Autodesk Inventor part; units mm, degrees
(part 3 of 3)
  spline S428 degree 2 poles (88.3492, 102.9904) (88.3492, 103.2264) (88.4685, 103.644) (88.7097, 103.9578) (89.0676, 104.1394) (89.3062, 104.1394) knots 0 0 0 1 2 3 4 4 4
  spline S429 degree 2 poles (89.3062, 104.1394) (89.3789, 104.1394) (89.5215, 104.1264) (89.5838, 104.1057) knots 0 0 0 1 2 2 2
  line L489 (89.5838, 104.1057) -> (89.7757, 103.8204)
  line L490 (89.7757, 103.8204) -> (89.7757, 104.1446)
  line L491 (89.7757, 104.1446) -> (90.1569, 104.1057)
  line L492 (90.1569, 104.1057) -> (90.1569, 101.8052)
  spline S430 degree 2 poles (90.1569, 101.8052) (90.1569, 101.6081) (90.0221, 101.2631) (89.7705, 101.0064) (89.4048, 100.8585) (89.1766, 100.8585) knots 0 0 0 1 2 3 4 4 4
  spline S431 degree 2 poles (89.1766, 100.8585) (89.0184, 100.8585) (88.7798, 100.9389) (88.6942, 100.9882) knots 0 0 0 1 2 2 2
  spline S432 degree 2 poles (88.6942, 100.9882) (88.5982, 101.0427) (88.5282, 101.1179) knots 0 0 0 1 1 1
  line L493 (88.5282, 101.1179) -> (88.7253, 101.3383)
  spline S433 degree 2 poles (88.7253, 101.3383) (88.7823, 101.2943) (88.855, 101.2579) knots 0 0 0 1 1 1
  spline S434 degree 2 poles (88.855, 101.2579) (88.9172, 101.2294) (89.0832, 101.1801) (89.1792, 101.1801) knots 0 0 0 1 2 2 2
  spline S435 degree 2 poles (89.1792, 101.1801) (89.3036, 101.1801) (89.5215, 101.2839) (89.6823, 101.4602) (89.7757, 101.6989) (89.7757, 101.8337) knots 0 0 0 1 2 3 4 4 4
  line L494 (89.7757, 101.8337) -> (89.7757, 102.1683)
  spline S436 degree 2 poles (89.7757, 103.5714) (89.7212, 103.6388) (89.6486, 103.6933) knots 0 0 0 1 1 1
  spline S437 degree 2 poles (89.6486, 103.6933) (89.5863, 103.74) (89.41, 103.8178) (89.2959, 103.8178) knots 0 0 0 1 2 2 2
  spline S438 degree 2 poles (89.2959, 103.8178) (89.174, 103.8178) (88.9976, 103.7426) (88.8705, 103.6129) (88.7927, 103.4417) (88.746, 103.2524) (88.7305, 103.0579) (88.7305, 102.9671) knots 0 0 0 1 2 3 4 5 6 6 6
  spline S439 degree 2 poles (88.7305, 102.9671) (88.7305, 102.7959) (88.8057, 102.5106) (88.9406, 102.3031) (89.1299, 102.1864) (89.244, 102.1864) knots 0 0 0 1 2 3 4 4 4
  spline S440 degree 2 poles (89.244, 102.1864) (89.3477, 102.1864) (89.5085, 102.2305) (89.6382, 102.3057) (89.7368, 102.3991) (89.7757, 102.4484) knots 0 0 0 1 2 3 4 4 4
  line L495 (89.7757, 102.4484) -> (89.7757, 103.5714)
  line L496 (92.1851, 104.1057) -> (92.5663, 104.1446)
  line L497 (92.5663, 104.1446) -> (92.5663, 101.896)
  line L498 (92.5663, 101.896) -> (92.1851, 101.896)
  line L499 (92.1851, 101.896) -> (92.1851, 102.2227)
  line L500 (92.1851, 102.2227) -> (92.0632, 102.0101)
  spline S441 degree 2 poles (92.0632, 102.0101) (92.0269, 101.9841) (91.9283, 101.9323) (91.8038, 101.8908) (91.656, 101.8622) (91.573, 101.8622) knots 0 0 0 1 2 3 4 4 4
  spline S442 degree 2 poles (91.573, 101.8622) (91.4122, 101.8622) (91.1814, 101.979) (91.0335, 102.1864) (90.9609, 102.4743) (90.9609, 102.6429) knots 0 0 0 1 2 3 4 4 4
  line L501 (90.9609, 102.6429) -> (90.9609, 104.1057)
  line L502 (90.9609, 104.1057) -> (91.3422, 104.1446)
  line L503 (91.3422, 104.1446) -> (91.3422, 102.6429)
  spline S443 degree 2 poles (91.3422, 102.6429) (91.3422, 102.4276) (91.5159, 102.1838) (91.7027, 102.1838) knots 0 0 0 1 2 2 2
  spline S444 degree 2 poles (91.7027, 102.1838) (91.7727, 102.1838) (91.905, 102.2279) (92.0295, 102.2954) (92.1384, 102.3758) (92.1851, 102.4147) knots 0 0 0 1 2 3 4 4 4
  line L504 (92.1851, 102.4147) -> (92.1851, 104.1057)
  line L505 (93.7516, 101.896) -> (93.3703, 101.896)
  line L506 (93.3703, 101.896) -> (93.3703, 104.0149)
  line L507 (93.3703, 104.0149) -> (93.7516, 104.0564)
  line L508 (93.7516, 104.0564) -> (93.7516, 101.896)
  line L509 (93.3573, 104.9071) -> (93.7645, 104.9071)
  line L510 (93.7645, 104.9071) -> (93.7645, 104.5051)
  line L511 (93.7645, 104.5051) -> (93.3573, 104.5051)
  line L512 (93.3573, 104.5051) -> (93.3573, 104.9071)
  line L513 (95.7979, 101.896) -> (95.7979, 102.2202)
  line L514 (95.7979, 102.2202) -> (95.6059, 101.9945)
  spline S445 degree 2 poles (95.6059, 101.9945) (95.5722, 101.9712) (95.4866, 101.9219) (95.3829, 101.8856) (95.2558, 101.8622) (95.178, 101.8622) knots 0 0 0 1 2 3 4 4 4
  spline S446 degree 2 poles (95.178, 101.8622) (95.012, 101.8622) (94.7267, 102.0256) (94.5167, 102.3135) (94.3948, 102.7129) (94.3948, 102.9515) knots 0 0 0 1 2 3 4 4 4
  spline S447 degree 2 poles (94.3948, 102.9515) (94.3948, 103.1927) (94.5504, 103.6129) (94.8357, 103.9241) (95.2377, 104.1031) (95.4866, 104.1031) knots 0 0 0 1 2 3 4 4 4
  line L515 (95.4866, 104.1031) -> (95.7979, 104.1031)
  line L516 (95.7979, 104.1031) -> (95.7979, 105.1483)
  line L517 (95.7979, 105.1483) -> (96.1791, 105.1094)
  line L518 (96.1791, 105.1094) -> (96.1791, 102.2565)
  line L519 (96.1791, 102.2565) -> (96.218, 101.896)
  line L520 (96.218, 101.896) -> (95.7979, 101.896)
  spline S448 degree 2 poles (95.4892, 103.7815) (95.3051, 103.7815) (95.0354, 103.644) (94.859, 103.408) (94.776, 103.0864) (94.776, 102.9048) knots 0 0 0 1 2 3 4 4 4
  spline S449 degree 2 poles (94.776, 102.9048) (94.776, 102.7259) (94.859, 102.4562) (94.9939, 102.2772) (95.1676, 102.1864) (95.2558, 102.1864) knots 0 0 0 1 2 3 4 4 4
  spline S450 degree 2 poles (95.2558, 102.1864) (95.3518, 102.1864) (95.5126, 102.2513) (95.65, 102.3472) (95.759, 102.4614) (95.7979, 102.5106) knots 0 0 0 1 2 3 4 4 4
  line L521 (95.7979, 102.5106) -> (95.7979, 103.7815)
  line L522 (95.7979, 103.7815) -> (95.4892, 103.7815)
  spline S451 degree 2 poles (98.5185, 102.1553) (98.4562, 102.0905) (98.3084, 101.9841) (98.1269, 101.9037) (97.909, 101.8622) (97.7741, 101.8622) knots 0 0 0 1 2 3 4 4 4
  spline S452 degree 2 poles (97.7741, 101.8622) (97.507, 101.8622) (97.1309, 102.0516) (96.8923, 102.368) (96.7808, 102.7778) (96.7808, 103.0008) knots 0 0 0 1 2 3 4 4 4
  spline S453 degree 2 poles (96.7808, 103.0008) (96.7808, 103.1435) (96.8327, 103.4236) (96.9364, 103.6751) (97.0946, 103.893) (97.3021, 104.0486) (97.5667, 104.1394) (97.7249, 104.1394) knots 0 0 0 1 2 3 4 5 6 6 6
  spline S454 degree 2 poles (97.7249, 104.1394) (97.9401, 104.1394) (98.2591, 103.9993) (98.4666, 103.7452) (98.5678, 103.3924) (98.5678, 103.1772) knots 0 0 0 1 2 3 4 4 4
  spline S455 degree 2 poles (98.5678, 103.1772) (98.5678, 103.1149) (98.56, 102.9671) (98.5522, 102.8997) knots 0 0 0 1 2 2 2
  line L523 (98.5522, 102.8997) -> (97.1621, 102.8997)
  spline S456 degree 2 poles (97.1621, 102.8997) (97.1621, 102.7492) (97.2451, 102.4899) (97.3929, 102.2954) (97.603, 102.1838) (97.7352, 102.1838) knots 0 0 0 1 2 3 4 4 4
  spline S457 degree 2 poles (97.7352, 102.1838) (97.8623, 102.1838) (98.0542, 102.2227) (98.1891, 102.2772) (98.2773, 102.3317) (98.3006, 102.3472) knots 0 0 0 1 2 3 4 4 4
  line L524 (98.3006, 102.3472) -> (98.5185, 102.1553)
  spline S458 degree 2 poles (98.1865, 103.2005) (98.1891, 103.2239) (98.1917, 103.2679) (98.1917, 103.2887) knots 0 0 0 1 2 2 2
  spline S459 degree 2 poles (98.1917, 103.2887) (98.1917, 103.4028) (98.1372, 103.5973) (98.0309, 103.74) (97.8675, 103.8204) (97.7534, 103.8204) knots 0 0 0 1 2 3 4 4 4
  spline S460 degree 2 poles (97.7534, 103.8204) (97.6211, 103.8204) (97.4292, 103.7348) (97.2995, 103.5999) (97.2191, 103.4391) (97.201, 103.3665) knots 0 0 0 1 2 3 4 4 4
  line L525 (97.201, 103.3665) -> (97.0946, 103.146)
  line L526 (97.0946, 103.146) -> (97.4525, 103.2005)
  line L527 (97.4525, 103.2005) -> (98.1865, 103.2005)
  point P0 (0, 65.2863)
  constraints: 2 other
emboss "Emboss1" sketch "Sketch3" operation cut depth 1 direction (0, -1, 0)
sketch "Sketch4" plane through (4.953, 113.8555, 65.2863) normal (0, 0, 1) x (1, 0, 0)
  line L0 (0, 0) -> (120.894, 0) construction
  line L1 (120.894, -16.552) -> (0, -16.552) construction
  line L2 (0, 0) -> (120.894, -16.552) construction
  point P0 (-4.953, -113.8555)
  point P1 (60.447, -8.276)
  point P2 (60.447, -8.276)
  constraints: 2 end point, 1 coincident, 1 midpoint
hole "Hole1" at (65.4, 105.5795, 65.2863) direction (0, 0, -1) diameter 6.35 end through all
sketch "Sketch5" plane through (0, 0, 0) normal (0, 0, 1) x (1, 0, 0)
  circle A0 centre (65.4, 105.5795) radius 3.175 construction
  circle A1 centre (65.4, 105.5795) radius 6.35
  point P0 (0, 0)
  dimension "d23" = 12.7
  constraints: 1 centre point, 1 coincident
  measures "d23" diameter of A1
extrude "Extrusion3" cut sketch "Sketch5" along normal mid plane 100
equation "\"d0\" = hull_od"
equation "\"hull_od\" = 219.075"
equation "\"hull_id\" = 201.7268"
equation "\"hull_wall\" = 8.6741"
equation "\"hull_length\" = 609.6"
equation "\"hull_spacing\" = 390.525"
equation "\"impeller_od\" = 76.2"
equation "\"impeller_clearance\" = 0.5"
equation "\"impeller_shaft_id\" = 3.175"
equation "\"impeller_shaft_od\" = 5.715"
equation "\"impeller_shaft_support\" = 3.175"
equation "\"impeller_intake_od\" = 19.05"
equation "\"impeller_vane_thick\" = 2"
equation "\"impeller_vane_inner_rad\" = 3.175"
equation "\"impeller_vane_outer_rad\" = 0.37206"
equation "\"magnet_od\" = 5.95"
equation "\"magnet_clearance\" = 0.25"
equation "\"magnet_rad\" = 0.25"
equation "\"magnet_circle_offset\" = 3.175"
equation "\"motor_shaft_od\" = 12.7"
equation "\"motor_shaft_length\" = 31.75"
equation "\"motor_shaft_key\" = 3.048"
equation "\"slab_thick\" = 34.671"
body "Solid1"
